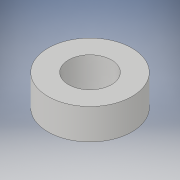
# Autodesk Inventor part: Spacer 3mm
Saved by Autodesk Inventor 2019 (Build 230136000, 136)
## iProperties
Created: 2019-02-04
Part Number: Spacer 3mm
Material: Generic
Document SubType Name: Modeling
Designer: mrhftc
Density: 1 g/cm^3
Appearance: Default
Author: mrhftc
Autodesk Inventor part; units mm, degrees
ref_plane "YZ Plane" through (0, 0, 0) normal (1, 0, 0) x (0, 1, 0)
ref_plane "XZ Plane" through (0, 0, 0) normal (0, 1, 0) x (-1, 0, 0)
ref_plane "XY Plane" through (0, 0, 0) normal (0, 0, 1) x (1, 0, 0)
sketch "Sketch1" plane through (0, 0, 0) normal (0, 1, 0) x (-1, 0, 0)
  circle A0 centre (18.2147, 57.8222) radius 2.1
  circle A1 centre (18.2147, 57.8222) radius 4.1
  point P0 (0, 0)
  dimension "d0" = 4.2
  dimension "d1" = 2
  constraints: 2 centre point, 1 coincident
  measures "d0" diameter of A0
  measures "d1" radial gap between concentric circles of A0 A1
extrude "Extrusion1" add sketch "Sketch1" along normal blind 3.175
sketch "Sketch2" plane through (-18.2147, 3.175, 57.8222) normal (0, 1, 0) x (1, 0, 0)
  line L0 (-4.2917, 4.2453) -> (4.2078, 4.2453)
  line L1 (4.2078, 4.2453) -> (4.2078, -4.2223)
  line L2 (4.2078, -4.2223) -> (-4.2917, -4.2223)
  line L3 (-4.2917, -4.2223) -> (-4.2917, 4.2453)
  point P0 (18.2147, 57.8222)
  constraints: 8 end point, 2 parallel, 1 horizontal, 1 perpendicular
extrude "Extrusion2" cut sketch "Sketch2" against normal blind 0.175
body "Solid1"
